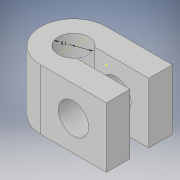
# Autodesk Inventor part: base and bar clamp
Saved by Autodesk Inventor 2018 (Build 220112000, 112)
## iProperties
Created: 2018-01-17
Part Number: base and bar clamp
Material: Generic
Document SubType Name: Modeling
Designer: junai
Density: 1 g/cm^3
Appearance: Default
Author: junai
Autodesk Inventor part; units mm, degrees
ref_plane "YZ Plane" through (0, 0, 0) normal (1, 0, 0) x (0, 1, 0)
ref_plane "XZ Plane" through (0, 0, 0) normal (0, 1, 0) x (-1, 0, 0)
ref_plane "XY Plane" through (0, 0, 0) normal (0, 0, 1) x (1, 0, 0)
sketch "Sketch1" plane through (0, 0, 0) normal (0, 1, 0) x (-1, 0, 0)
  point P0 (0, 0)
sketch "Sketch2" plane through (0, 0, 0) normal (0, 1, 0) x (-1, 0, 0)
  point P0 (0, 0)
sketch "Sketch3" plane through (0, 0, 0) normal (0, 1, 0) x (-1, 0, 0)
  line L0 (0, 0) -> (0, -8.75) construction
  line L1 (0, 0) -> (0, 8.75) construction
  line L2 (8.75, 8.75) -> (-8.75, 8.75)
  line L3 (-8.75, 8.75) -> (-8.75, -8.75)
  line L4 (-8.75, -8.75) -> (8.75, -8.75)
  line L5 (8.75, -8.75) -> (8.75, 8.75)
  circle A0 centre (8.75, 0) radius 8.75
  circle A1 centre (8.75, 0) radius 4.05
  line L6 (0, 0) -> (4.05, 0) construction
  dimension "d0" = 8.75
  dimension "d1" = 8.75
  dimension "d2" = 17.5
  dimension "d3" = 17.5
  dimension "d7" = 8.1
  dimension "d9" = 4.05
  constraints: 14 end point, 3 midpoint, 2 centre point, 2 coincident, 2 horizontal, 2 parallel, 2 vertical, 1 perpendicular
  measures "d0" distance of L0.end L0.start
  measures "d1" distance of L1.end L0.start
  measures "d2" distance of L4.end L3.end
  measures "d3" diameter of A0
  measures "d7" diameter of A1
  measures "d9" distance of L0.start L6.end
sketch "Sketch4" plane through (0, 0, 0) normal (0, 1, 0) x (-1, 0, 0)
  point P0 (0, 0)
sketch "Sketch5" plane through (0, 0, 0) normal (0, 1, 0) x (-1, 0, 0)
  point P0 (0, 0)
extrude "Extrusion2" add sketch "Sketch3" against normal blind 16 contours A0 L4 L3 L2 | A0 L5 A1 | L5 A1 A0 | L5 A1 picked at (7.639, -0.7669)
sketch "Sketch6" plane through (0, 0, 0) normal (0, 1, 0) x (1, 0, 0)
  line L0 (-8.75, 4.05) -> (-8.75, -4.05) projected
  circle A0 centre (-8.75, 0) radius 4.05
  point P0 (0, 0)
  constraints: 1 centre point, 1 midpoint
sketch "Sketch7" plane through (0, 0, 0) normal (0, 1, 0) x (1, 0, 0)
  line L0 (-8.75, 4.05) -> (-8.75, -4.05) construction
  circle A0 centre (-8.75, 0) radius 4.05 construction
  arc A1 (-8.75, 4.05) -> (-8.75, -4.05) centre (-8.75, 0) ccw construction
  arc A2 (-8.75, 8.75) -> (-8.75, -8.75) centre (-8.75, 0) ccw construction
  point P0 (0, 0)
  dimension "d12" = 8.1
  constraints: 2 concentric, 1 centre point, 1 midpoint
  measures "d12" diameter of A0
extrude "Extrusion3" cut sketch "Sketch6" against normal blind 16
sketch "Sketch8" plane through (-8.75, 0, 8.75) normal (0, 0, 1) x (1, 0, 0)
  line L0 (17.5, -16) -> (0, -16) construction
  line L1 (8.75, -16) -> (8.75, 0) construction
  circle A0 centre (8.75, -8) radius 4.05
  dimension "d15" = 8.1
  constraints: 2 end point, 2 midpoint, 1 centre point, 1 coincident, 1 vertical
  measures "d15" diameter of A0
extrude "Extrusion4" cut sketch "Sketch8" against normal up to next
sketch "Sketch9" plane through (0, 0, 0) normal (0, 1, 0) x (1, 0, 0)
  point P0 (0, 0)
sketch "Sketch10" plane through (0, 0, 0) normal (0, 1, 0) x (1, 0, 0)
  point P0 (0, 0)
sketch "Sketch11" plane through (0, 0, 0) normal (0, 1, 0) x (1, 0, 0)
  point P0 (0, 0)
sketch "Sketch12" plane through (0, 0, 0) normal (0, 1, 0) x (1, 0, 0)
  line L0 (8.75, 8.75) -> (8.75, -8.75) construction
  line L1 (8.75, 8.75) -> (8.75, 2.5) construction
  line L2 (8.75, 2.5) -> (8.75, -2.5) construction
  line L3 (8.75, -2.5) -> (8.75, -8.75) construction
  circle A0 centre (-8.75, 0) radius 4.05 projected
  line L4 (8.75, -2.5) -> (-5.5637, -2.5)
  line L5 (-5.5637, -2.5) -> (-5.5637, 2.5)
  line L6 (-5.5637, 2.5) -> (8.75, 2.5)
  line L7 (8.75, 2.5) -> (8.75, -2.5)
  point P0 (0, 0)
  dimension "d18" = 6.25
  dimension "d19" = 5
  dimension "d20" = 6.25
  constraints: 14 end point, 3 point on line, 2 parallel, 1 collinear, 1 horizontal, 1 perpendicular, 2 other
  measures "d18" distance of L0.start L1.end
  measures "d19" distance of L1.end L2.end
  measures "d20" distance of L2.end L0.end
extrude "Extrusion5" cut sketch "Sketch12" against normal up to next contours A0 L5 | A0 L6 L7 L4 picked at (-5.4064, -0.5793)
body "Solid2"
